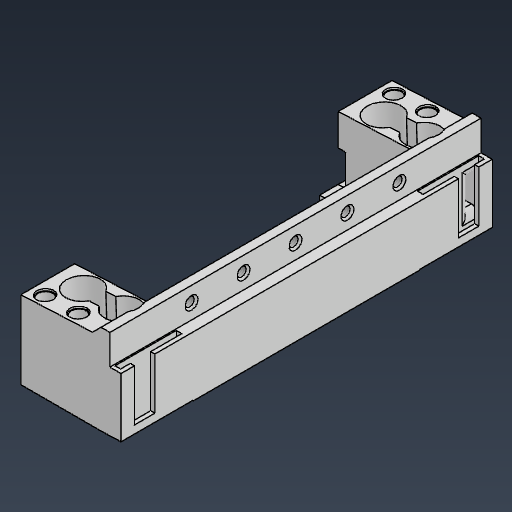
# Autodesk Inventor part: FonrtMount
Saved by Autodesk Inventor 2026.2 (Build 302298010, 298A)
## iProperties
Created: 2026-04-04
Part Number: FonrtMount
Material: Generic
Document SubType Name: Modeling
Designer: szymo
Density: 1 g/cm^3
Appearance: Default
Author: szymo
Autodesk Inventor part; units mm, degrees
(part 1 of 2)
ref_plane "YZ Plane" through (0, 0, 0) normal (1, 0, 0) x (0, 1, 0)
ref_plane "XZ Plane" through (0, 0, 0) normal (0, 1, 0) x (-1, 0, 0)
ref_plane "XY Plane" through (0, 0, 0) normal (0, 0, 1) x (1, 0, 0)
sketch "Sketch1" plane through (0, 0, 0) normal (0, 0, 1) x (1, 0, 0)
  line L0 (-27, 86.2958) -> (-6.5, 86.2958) projected
  line L1 (-6.5, 86.2958) -> (-6.5, 69.7958) projected
  line L2 (-27, 69.7958) -> (-6.5, 69.7958) projected
  line L3 (-27, 86.2958) -> (-27, 69.7958) projected
  line L4 (0, 94.9) -> (0, 81.9) projected
  line L5 (0, 81.9) -> (-3, 81.9) projected
  line L6 (-3, 81.9) -> (-3, 89.9) projected
  line L7 (-3, 89.9) -> (-5, 89.9) projected
  line L8 (-5, 89.9) -> (0, 94.9) projected
  circle A0 centre (-14.5, 55.2958) radius 14.5 projected
  line L9 (-8.2042, 86.6958) -> (-6, 86.6958)
  line L10 (-6, 86.6958) -> (-6, 69.2958)
  line L11 (-6, 69.2958) -> (-10.7251, 69.2958)
  line L12 (-4, 65.2958) -> (0, 65.2958)
  line L13 (0, 65.2958) -> (0, 81.4)
  line L14 (0, 81.4) -> (-3, 81.4)
  line L15 (-3, 81.4) -> (-3, 89.5)
  line L16 (-5.4, 89.5) -> (-8.2042, 86.6958)
  line L17 (-5.4, 89.5) -> (-3, 89.5)
  line L18 (-5.4, 89.5) -> (-5, 89.9) construction
  line L19 (-9.2085, 69.2958) -> (-9.2085, 68.7958)
  line L20 (-7.7042, 87.1958) -> (-7.7042, 86.6958)
  arc A1 (-19.3741, 42.1797) -> (-18.7931, 40.8751) centre (-13.6387, 43.9522) ccw construction
  arc A2 (-18.9897, 42.5035) -> (-19.3741, 42.1797) centre (-13, 35.0012) ccw construction
  arc A3 (-17.8029, 41.709) -> (-18.9897, 42.5035) centre (-21.712, 37.1532) ccw construction
  arc A4 (-17.4452, 41.9512) -> (-17.8029, 41.709) centre (-13, 35.0012) ccw construction
  arc A5 (-17.7423, 43.3481) -> (-17.4452, 41.9512) centre (-11.7637, 43.8894) ccw construction
  arc A6 (-17.299, 43.5848) -> (-17.7423, 43.3481) centre (-13, 35.0012) ccw construction
  arc A7 (-16.3033, 42.561) -> (-17.299, 43.5848) centre (-21.0742, 38.9175) ccw construction
  arc A8 (-15.9031, 42.7235) -> (-16.3033, 42.561) centre (-13, 35.0012) ccw construction
  arc A9 (-15.9033, 44.1517) -> (-15.9031, 42.7235) centre (-9.9428, 43.4382) ccw construction
  arc A10 (-15.4204, 44.2911) -> (-15.9033, 44.1517) centre (-13, 35.0012) ccw construction
  arc A11 (-14.6593, 43.0826) -> (-15.4204, 44.2911) centre (-20.0835, 40.5106) ccw construction
  arc A12 (-14.2341, 43.1584) -> (-14.6593, 43.0826) centre (-13, 35.0012) ccw construction
  arc A13 (-13.9373, 44.5553) -> (-14.2341, 43.1584) centre (-8.2554, 42.6182) ccw construction
  arc A14 (-13.436, 44.5913) -> (-13.9373, 44.5553) centre (-13, 35.0012) ccw construction
  arc A15 (-12.9429, 43.251) -> (-13.436, 44.5913) centre (-18.7832, 41.8629) ccw construction
  arc A16 (-12.5112, 43.2367) -> (-12.9429, 43.251) centre (-13, 35.0012) ccw construction
  arc A17 (-11.9304, 44.5414) -> (-12.5112, 43.2367) centre (-6.7755, 41.4653) ccw construction
  arc A18 (-11.4326, 44.4724) -> (-11.9304, 44.5414) centre (-13, 35.0012) ccw construction
  arc A19 (-11.2289, 43.0588) -> (-11.4326, 44.4724) centre (-17.2302, 42.9154) ccw construction
  arc A20 (-10.8096, 42.9551) -> (-11.2289, 43.0588) centre (-13, 35.0012) ccw construction
  arc A21 (-9.9703, 44.1106) -> (-10.8096, 42.9551) centre (-5.5675, 40.0299) ccw construction
  arc A22 (-9.4977, 43.9395) -> (-9.9703, 44.1106) centre (-13, 35.0012) ccw construction
  arc A23 (-9.5923, 42.5145) -> (-9.4977, 43.9395) centre (-15.4923, 43.622) ccw construction
  arc A24 (-9.2038, 42.3259) -> (-9.5923, 42.5145) centre (-13, 35.0012) ccw construction
  arc A25 (-8.1425, 43.2816) -> (-9.2038, 42.3259) centre (-4.6844, 38.3747) ccw construction
  arc A26 (-7.7158, 43.016) -> (-8.1425, 43.2816) centre (-13, 35.0012) ccw construction
  arc A27 (-8.1047, 41.6418) -> (-7.7158, 43.016) centre (-13.6455, 43.9518) ccw construction
  arc A28 (-7.7638, 41.3765) -> (-8.1047, 41.6418) centre (-13, 35.0012) ccw construction
  arc A29 (-6.5271, 42.0907) -> (-7.7638, 41.3765) centre (-4.1648, 36.572) ccw construction
  arc A30 (-6.1649, 41.7423) -> (-6.5271, 42.0907) centre (-13, 35.0012) ccw construction
  arc A31 (-6.831, 40.4789) -> (-6.1649, 41.7423) centre (-11.7705, 43.8904) ccw construction
  arc A32 (-6.5527, 40.1486) -> (-6.831, 40.4789) centre (-13, 35.0012) ccw construction
  arc A33 (-5.1945, 40.59) -> (-6.5527, 40.1486) centre (-4.0312, 34.7008) ccw construction
  arc A34 (-4.9127, 40.1739) -> (-5.1945, 40.59) centre (-13, 35.0012) ccw construction
  arc A35 (-5.8269, 39.0766) -> (-4.9127, 40.1739) centre (-9.9492, 43.4405) ccw construction
  arc A36 (-5.6234, 38.6956) -> (-5.8269, 39.0766) centre (-13, 35.0012) ccw construction
  arc A37 (-4.2031, 38.845) -> (-5.6234, 38.6956) centre (-4.2897, 32.8426) ccw construction
  arc A38 (-4.014, 38.3794) -> (-4.2031, 38.845) centre (-13, 35.0012) ccw construction
  arc A39 (-5.1363, 37.4962) -> (-4.014, 38.3794) centre (-8.2612, 42.6218) ccw construction
  arc A40 (-5.0165, 37.0812) -> (-5.1363, 37.4962) centre (-13, 35.0012) ccw construction
  arc A41 (-3.5962, 36.9321) -> (-5.0165, 37.0812) centre (-4.9288, 31.0788) ccw construction
  arc A42 (-3.508, 36.4373) -> (-3.5962, 36.9321) centre (-13, 35.0012) ccw construction
  arc A43 (-4.7894, 35.8067) -> (-3.508, 36.4373) centre (-6.7804, 41.47) ccw construction
  arc A44 (-4.7585, 35.3759) -> (-4.7894, 35.8067) centre (-13, 35.0012) ccw construction
  arc A45 (-3.4002, 34.9347) -> (-4.7585, 35.3759) centre (-5.9207, 29.4864) ccw construction
  arc A46 (-3.4169, 34.4324) -> (-3.4002, 34.9347) centre (-13, 35.0012) ccw construction
  arc A47 (-4.8014, 34.082) -> (-3.4169, 34.4324) centre (-5.5713, 40.0355) ccw construction
  arc A48 (-4.8607, 33.6542) -> (-4.8014, 34.082) centre (-13, 35.0012) ccw construction
  arc A49 (-3.6238, 32.9403) -> (-4.8607, 33.6542) centre (-7.222, 28.1351) ccw construction
  arc A50 (-3.7445, 32.4524) -> (-3.6238, 32.9403) centre (-13, 35.0012) ccw construction
  arc A51 (-5.1716, 32.3975) -> (-3.7445, 32.4524) centre (-4.687, 38.381) ccw construction
  arc A52 (-5.3186, 31.9914) -> (-5.1716, 32.3975) centre (-13, 35.0012) ccw construction
  arc A53 (-4.2572, 31.0359) -> (-5.3186, 31.9914) centre (-8.7758, 27.0838) ccw construction
  arc A54 (-4.4767, 30.5838) -> (-4.2572, 31.0359) centre (-13, 35.0012) ccw construction
  arc A55 (-5.884, 30.8268) -> (-4.4767, 30.5838) centre (-4.1659, 36.5788) ccw construction
  arc A56 (-6.1122, 30.4601) -> (-5.884, 30.8268) centre (-13, 35.0012) ccw construction
  arc A57 (-5.2727, 29.3048) -> (-6.1122, 30.4601) centre (-10.5142, 26.3786) ccw construction
  arc A58 (-5.5814, 28.9082) -> (-5.2727, 29.3048) centre (-13, 35.0012) ccw construction
  arc A59 (-6.9074, 29.4385) -> (-5.5814, 28.9082) centre (-4.031, 34.7076) ccw construction
  arc A60 (-7.2069, 29.1273) -> (-6.9074, 29.4385) centre (-13, 35.0012) ccw construction
  arc A61 (-6.6259, 27.8227) -> (-7.2069, 29.1273) centre (-12.3613, 26.0502) ccw construction
  arc A62 (-7.0103, 27.4989) -> (-6.6259, 27.8227) centre (-13, 35.0012) ccw construction
  arc A63 (-8.1971, 28.2934) -> (-7.0103, 27.4989) centre (-4.288, 32.8492) ccw construction
  arc A64 (-8.5548, 28.0512) -> (-8.1971, 28.2934) centre (-13, 35.0012) ccw construction
  arc A65 (-8.2577, 26.6543) -> (-8.5548, 28.0512) centre (-14.2363, 26.113) ccw construction
  arc A66 (-8.701, 26.4176) -> (-8.2577, 26.6543) centre (-13, 35.0012) ccw construction
  arc A67 (-9.6967, 27.4414) -> (-8.701, 26.4176) centre (-4.9258, 31.0849) ccw construction
  arc A68 (-10.0969, 27.2789) -> (-9.6967, 27.4414) centre (-13, 35.0012) ccw construction
  arc A69 (-10.0967, 25.8507) -> (-10.0969, 27.2789) centre (-16.0572, 26.5642) ccw construction
  arc A70 (-10.5796, 25.7113) -> (-10.0967, 25.8507) centre (-13, 35.0012) ccw construction
  arc A71 (-11.3407, 26.9198) -> (-10.5796, 25.7113) centre (-5.9165, 29.4918) ccw construction
  arc A72 (-11.7659, 26.844) -> (-11.3407, 26.9198) centre (-13, 35.0012) ccw construction
  arc A73 (-12.0627, 25.4471) -> (-11.7659, 26.844) centre (-17.7446, 27.3842) ccw construction
  arc A74 (-12.564, 25.4111) -> (-12.0627, 25.4471) centre (-13, 35.0012) ccw construction
  arc A75 (-13.0571, 26.7514) -> (-12.564, 25.4111) centre (-7.2168, 28.1395) ccw construction
  arc A76 (-13.4888, 26.7657) -> (-13.0571, 26.7514) centre (-13, 35.0012) ccw construction
  arc A77 (-14.0696, 25.461) -> (-13.4888, 26.7657) centre (-19.2245, 28.5371) ccw construction
  arc A78 (-14.5674, 25.53) -> (-14.0696, 25.461) centre (-13, 35.0012) ccw construction
  arc A79 (-14.7711, 26.9436) -> (-14.5674, 25.53) centre (-8.7698, 27.087) ccw construction
  arc A80 (-15.1904, 27.0473) -> (-14.7711, 26.9436) centre (-13, 35.0012) ccw construction
  arc A81 (-16.0297, 25.8918) -> (-15.1904, 27.0473) centre (-20.4325, 29.9725) ccw construction
  arc A82 (-16.5023, 26.0629) -> (-16.0297, 25.8918) centre (-13, 35.0012) ccw construction
  arc A83 (-16.4077, 27.4879) -> (-16.5023, 26.0629) centre (-10.5077, 26.3804) ccw construction
  arc A84 (-16.7962, 27.6765) -> (-16.4077, 27.4879) centre (-13, 35.0012) ccw construction
  arc A85 (-17.8575, 26.7208) -> (-16.7962, 27.6765) centre (-21.3156, 31.6277) ccw construction
  arc A86 (-18.2842, 26.9864) -> (-17.8575, 26.7208) centre (-13, 35.0012) ccw construction
  arc A87 (-17.8953, 28.3605) -> (-18.2842, 26.9864) centre (-12.3545, 26.0506) ccw construction
  arc A88 (-18.2362, 28.6259) -> (-17.8953, 28.3605) centre (-13, 35.0012) ccw construction
  arc A89 (-19.4729, 27.9117) -> (-18.2362, 28.6259) centre (-21.8352, 33.4304) ccw construction
  arc A90 (-19.8351, 28.2601) -> (-19.4729, 27.9117) centre (-13, 35.0012) ccw construction
  arc A91 (-19.169, 29.5235) -> (-19.8351, 28.2601) centre (-14.2295, 26.112) ccw construction
  arc A92 (-19.4473, 29.8538) -> (-19.169, 29.5235) centre (-13, 35.0012) ccw construction
  arc A93 (-20.8055, 29.4124) -> (-19.4473, 29.8538) centre (-21.9688, 35.3016) ccw construction
  arc A94 (-21.0873, 29.8285) -> (-20.8055, 29.4124) centre (-13, 35.0012) ccw construction
  arc A95 (-20.1731, 30.9258) -> (-21.0873, 29.8285) centre (-16.0508, 26.5619) ccw construction
  arc A96 (-20.3766, 31.3068) -> (-20.1731, 30.9258) centre (-13, 35.0012) ccw construction
  arc A97 (-21.7969, 31.1574) -> (-20.3766, 31.3068) centre (-21.7103, 37.1598) ccw construction
  arc A98 (-21.986, 31.623) -> (-21.7969, 31.1574) centre (-13, 35.0012) ccw construction
  arc A99 (-20.8637, 32.5062) -> (-21.986, 31.623) centre (-17.7388, 27.3806) ccw construction
  arc A100 (-20.9835, 32.9212) -> (-20.8637, 32.5062) centre (-13, 35.0012) ccw construction
  arc A101 (-22.4038, 33.0703) -> (-20.9835, 32.9212) centre (-21.0712, 38.9236) ccw construction
  arc A102 (-22.492, 33.5651) -> (-22.4038, 33.0703) centre (-13, 35.0012) ccw construction
  arc A103 (-21.2106, 34.1957) -> (-22.492, 33.5651) centre (-19.2196, 28.5324) ccw construction
  arc A104 (-21.2415, 34.6265) -> (-21.2106, 34.1957) centre (-13, 35.0012) ccw construction
  arc A105 (-22.5998, 35.0677) -> (-21.2415, 34.6265) centre (-20.0793, 40.516) ccw construction
  arc A106 (-22.5831, 35.57) -> (-22.5998, 35.0677) centre (-13, 35.0012) ccw construction
  arc A107 (-21.1986, 35.9204) -> (-22.5831, 35.57) centre (-20.4287, 29.9669) ccw construction
  arc A108 (-21.1393, 36.3482) -> (-21.1986, 35.9204) centre (-13, 35.0012) ccw construction
  arc A109 (-22.3762, 37.0621) -> (-21.1393, 36.3482) centre (-18.778, 41.8673) ccw construction
  arc A110 (-22.2555, 37.55) -> (-22.3762, 37.0621) centre (-13, 35.0012) ccw construction
  arc A111 (-20.8284, 37.6049) -> (-22.2555, 37.55) centre (-21.313, 31.6214) ccw construction
  arc A112 (-20.6814, 38.011) -> (-20.8284, 37.6049) centre (-13, 35.0012) ccw construction
  arc A113 (-21.7428, 38.9665) -> (-20.6814, 38.011) centre (-17.2242, 42.9186) ccw construction
  arc A114 (-21.5233, 39.4186) -> (-21.7428, 38.9665) centre (-13, 35.0012) ccw construction
  arc A115 (-20.116, 39.1756) -> (-21.5233, 39.4186) centre (-21.8341, 33.4236) ccw construction
  arc A116 (-19.8878, 39.5423) -> (-20.116, 39.1756) centre (-13, 35.0012) ccw construction
  arc A117 (-20.7273, 40.6976) -> (-19.8878, 39.5423) centre (-15.4858, 43.6238) ccw construction
  arc A118 (-20.4186, 41.0942) -> (-20.7273, 40.6976) centre (-13, 35.0012) ccw construction
  arc A119 (-19.0926, 40.5639) -> (-20.4186, 41.0942) centre (-21.969, 35.2948) ccw construction
  arc A120 (-18.7931, 40.8751) -> (-19.0926, 40.5639) centre (-13, 35.0012) ccw construction
  circle A121 centre (-13, 35.0012) radius 9.6 construction
  line L21 (-4, 65.2958) -> (-27, 65.2958)
  line L22 (-27, 65.2958) -> (-27, 24.2538) construction
  line L23 (-27, 65.2958) -> (-27, 69.2958)
  line L24 (-27, 69.2958) -> (-9.2085, 69.2958)
  point P0 (0, 0)
  dimension "d0" = 4.5
  dimension "d1" = 0.5
  dimension "d2" = 0.5
  dimension "d3" = 0.4
  dimension "d4" = 45
  dimension "d5" = 0.4
  dimension "d6" = 0.5
  dimension "d11" = 0.5
  dimension "d12" = 0.5
  dimension "d32" = 2
  constraints: 32 end point, 7 perpendicular, 4 point on line, 3 horizontal, 3 point on circle, 3 vertical, 2 collinear, 1 coincident, 1 tangent, 3 other
  measures "d0" distance between parallel lines of L12 L2
  measures "d1" distance between parallel lines of L2 L11
  measures "d2" distance between parallel lines of L1 L10
  measures "d3" distance between parallel lines of L9 L0
  measures "d4" angle of L9 L16
  measures "d5" distance between parallel lines of L7 L17
  measures "d6" distance between parallel lines of L5 L14
  measures "d11" distance of L19.start L19.end
  measures "d12" distance of L20.start L20.end
  measures "d32" distance edge to line of A0 L22
extrude "Extrusion2" add sketch "Sketch1" along normal blind 19 and the other way blind 18.4 contours L19 L11 L10 L9 L20 L16 L17 L6 L15 L14 L13 L12 A0
sketch "Sketch2" plane through (0, 0, -18.4) normal (0, 0, -1) x (-1, 0, 0)
  arc A0 (18.7931, 40.8751) -> (19.3741, 42.1797) centre (13.6387, 43.9522) ccw construction
  arc A1 (19.3741, 42.1797) -> (18.9897, 42.5035) centre (13, 35.0012) ccw construction
  arc A2 (18.9897, 42.5035) -> (17.8029, 41.709) centre (21.712, 37.1532) ccw construction
  arc A3 (17.8029, 41.709) -> (17.4452, 41.9512) centre (13, 35.0012) ccw construction
  arc A4 (17.4452, 41.9512) -> (17.7423, 43.3481) centre (11.7637, 43.8894) ccw construction
  arc A5 (17.7423, 43.3481) -> (17.299, 43.5848) centre (13, 35.0012) ccw construction
  arc A6 (17.299, 43.5848) -> (16.3033, 42.561) centre (21.0742, 38.9175) ccw construction
  arc A7 (16.3033, 42.561) -> (15.9031, 42.7235) centre (13, 35.0012) ccw construction
  arc A8 (15.9031, 42.7235) -> (15.9033, 44.1517) centre (9.9428, 43.4382) ccw construction
  arc A9 (15.9033, 44.1517) -> (15.4204, 44.2911) centre (13, 35.0012) ccw construction
  arc A10 (15.4204, 44.2911) -> (14.6593, 43.0826) centre (20.0835, 40.5106) ccw construction
  arc A11 (14.6593, 43.0826) -> (14.2341, 43.1584) centre (13, 35.0012) ccw construction
  arc A12 (14.2341, 43.1584) -> (13.9373, 44.5553) centre (8.2554, 42.6182) ccw construction
  arc A13 (13.9373, 44.5553) -> (13.436, 44.5913) centre (13, 35.0012) ccw construction
  arc A14 (13.436, 44.5913) -> (12.9429, 43.251) centre (18.7832, 41.8629) ccw construction
  arc A15 (12.9429, 43.251) -> (12.5112, 43.2367) centre (13, 35.0012) ccw construction
  arc A16 (12.5112, 43.2367) -> (11.9304, 44.5414) centre (6.7755, 41.4653) ccw construction
  arc A17 (11.9304, 44.5414) -> (11.4326, 44.4724) centre (13, 35.0012) ccw construction
  arc A18 (11.4326, 44.4724) -> (11.2289, 43.0588) centre (17.2302, 42.9154) ccw construction
  arc A19 (11.2289, 43.0588) -> (10.8096, 42.9551) centre (13, 35.0012) ccw construction
  arc A20 (10.8096, 42.9551) -> (9.9703, 44.1106) centre (5.5675, 40.0299) ccw construction
  arc A21 (9.9703, 44.1106) -> (9.4977, 43.9395) centre (13, 35.0012) ccw construction
  arc A22 (9.4977, 43.9395) -> (9.5923, 42.5145) centre (15.4923, 43.622) ccw construction
  arc A23 (9.5923, 42.5145) -> (9.2038, 42.3259) centre (13, 35.0012) ccw construction
  arc A24 (9.2038, 42.3259) -> (8.1425, 43.2816) centre (4.6844, 38.3747) ccw construction
  arc A25 (8.1425, 43.2816) -> (7.7158, 43.016) centre (13, 35.0012) ccw construction
  arc A26 (7.7158, 43.016) -> (8.1047, 41.6418) centre (13.6455, 43.9518) ccw construction
  arc A27 (8.1047, 41.6418) -> (7.7638, 41.3765) centre (13, 35.0012) ccw construction
  arc A28 (7.7638, 41.3765) -> (6.5271, 42.0907) centre (4.1648, 36.572) ccw construction
  arc A29 (6.5271, 42.0907) -> (6.1649, 41.7423) centre (13, 35.0012) ccw construction
  arc A30 (6.1649, 41.7423) -> (6.831, 40.4789) centre (11.7705, 43.8904) ccw construction
  arc A31 (6.831, 40.4789) -> (6.5527, 40.1486) centre (13, 35.0012) ccw construction
  arc A32 (6.5527, 40.1486) -> (5.1945, 40.59) centre (4.0312, 34.7008) ccw construction
  arc A33 (5.1945, 40.59) -> (4.9127, 40.1739) centre (13, 35.0012) ccw construction
  arc A34 (4.9127, 40.1739) -> (5.8269, 39.0766) centre (9.9492, 43.4405) ccw construction
  arc A35 (5.8269, 39.0766) -> (5.6234, 38.6956) centre (13, 35.0012) ccw construction
  arc A36 (5.6234, 38.6956) -> (4.2031, 38.845) centre (4.2897, 32.8426) ccw construction
  arc A37 (4.2031, 38.845) -> (4.014, 38.3794) centre (13, 35.0012) ccw construction
  arc A38 (4.014, 38.3794) -> (5.1363, 37.4962) centre (8.2612, 42.6218) ccw construction
  arc A39 (5.1363, 37.4962) -> (5.0165, 37.0812) centre (13, 35.0012) ccw construction
  arc A40 (5.0165, 37.0812) -> (3.5962, 36.9321) centre (4.9288, 31.0788) ccw construction
  arc A41 (3.5962, 36.9321) -> (3.508, 36.4373) centre (13, 35.0012) ccw construction
  arc A42 (3.508, 36.4373) -> (4.7894, 35.8067) centre (6.7804, 41.47) ccw construction
  arc A43 (4.7894, 35.8067) -> (4.7585, 35.3759) centre (13, 35.0012) ccw construction
  arc A44 (4.7585, 35.3759) -> (3.4002, 34.9347) centre (5.9207, 29.4864) ccw construction
  arc A45 (3.4002, 34.9347) -> (3.4169, 34.4324) centre (13, 35.0012) ccw construction
  arc A46 (3.4169, 34.4324) -> (4.8014, 34.082) centre (5.5713, 40.0355) ccw construction
  arc A47 (4.8014, 34.082) -> (4.8607, 33.6542) centre (13, 35.0012) ccw construction
  arc A48 (4.8607, 33.6542) -> (3.6238, 32.9403) centre (7.222, 28.1351) ccw construction
  arc A49 (3.6238, 32.9403) -> (3.7445, 32.4524) centre (13, 35.0012) ccw construction
  arc A50 (3.7445, 32.4524) -> (5.1716, 32.3975) centre (4.687, 38.381) ccw construction
  arc A51 (5.1716, 32.3975) -> (5.3186, 31.9914) centre (13, 35.0012) ccw construction
  arc A52 (5.3186, 31.9914) -> (4.2572, 31.0359) centre (8.7758, 27.0838) ccw construction
  arc A53 (4.2572, 31.0359) -> (4.4767, 30.5838) centre (13, 35.0012) ccw construction
  arc A54 (4.4767, 30.5838) -> (5.884, 30.8268) centre (4.1659, 36.5788) ccw construction
  arc A55 (5.884, 30.8268) -> (6.1122, 30.4601) centre (13, 35.0012) ccw construction
  arc A56 (6.1122, 30.4601) -> (5.2727, 29.3048) centre (10.5142, 26.3786) ccw construction
  arc A57 (5.2727, 29.3048) -> (5.5814, 28.9082) centre (13, 35.0012) ccw construction
  arc A58 (5.5814, 28.9082) -> (6.9074, 29.4385) centre (4.031, 34.7076) ccw construction
  arc A59 (6.9074, 29.4385) -> (7.2069, 29.1273) centre (13, 35.0012) ccw construction
  arc A60 (7.2069, 29.1273) -> (6.6259, 27.8227) centre (12.3613, 26.0502) ccw construction
  arc A61 (6.6259, 27.8227) -> (7.0103, 27.4989) centre (13, 35.0012) ccw construction
  arc A62 (7.0103, 27.4989) -> (8.1971, 28.2934) centre (4.288, 32.8492) ccw construction
  arc A63 (8.1971, 28.2934) -> (8.5548, 28.0512) centre (13, 35.0012) ccw construction
  arc A64 (8.5548, 28.0512) -> (8.2577, 26.6543) centre (14.2363, 26.113) ccw construction
  arc A65 (8.2577, 26.6543) -> (8.701, 26.4176) centre (13, 35.0012) ccw construction
  arc A66 (8.701, 26.4176) -> (9.6967, 27.4414) centre (4.9258, 31.0849) ccw construction
  arc A67 (9.6967, 27.4414) -> (10.0969, 27.2789) centre (13, 35.0012) ccw construction
  arc A68 (10.0969, 27.2789) -> (10.0967, 25.8507) centre (16.0572, 26.5642) ccw construction
  arc A69 (10.0967, 25.8507) -> (10.5796, 25.7113) centre (13, 35.0012) ccw construction
  arc A70 (10.5796, 25.7113) -> (11.3407, 26.9198) centre (5.9165, 29.4918) ccw construction
  arc A71 (11.3407, 26.9198) -> (11.7659, 26.844) centre (13, 35.0012) ccw construction
  arc A72 (11.7659, 26.844) -> (12.0627, 25.4471) centre (17.7446, 27.3842) ccw construction
  arc A73 (12.0627, 25.4471) -> (12.564, 25.4111) centre (13, 35.0012) ccw construction
  arc A74 (12.564, 25.4111) -> (13.0571, 26.7514) centre (7.2168, 28.1395) ccw construction
  arc A75 (13.0571, 26.7514) -> (13.4888, 26.7657) centre (13, 35.0012) ccw construction
  arc A76 (13.4888, 26.7657) -> (14.0696, 25.461) centre (19.2245, 28.5371) ccw construction
  arc A77 (14.0696, 25.461) -> (14.5674, 25.53) centre (13, 35.0012) ccw construction
  arc A78 (14.5674, 25.53) -> (14.7711, 26.9436) centre (8.7698, 27.087) ccw construction
  arc A79 (14.7711, 26.9436) -> (15.1904, 27.0473) centre (13, 35.0012) ccw construction
  arc A80 (15.1904, 27.0473) -> (16.0297, 25.8918) centre (20.4325, 29.9725) ccw construction
  arc A81 (16.0297, 25.8918) -> (16.5023, 26.0629) centre (13, 35.0012) ccw construction
  arc A82 (16.5023, 26.0629) -> (16.4077, 27.4879) centre (10.5077, 26.3804) ccw construction
  arc A83 (16.4077, 27.4879) -> (16.7962, 27.6765) centre (13, 35.0012) ccw construction
  arc A84 (16.7962, 27.6765) -> (17.8575, 26.7208) centre (21.3156, 31.6277) ccw construction
  arc A85 (17.8575, 26.7208) -> (18.2842, 26.9864) centre (13, 35.0012) ccw construction
  arc A86 (18.2842, 26.9864) -> (17.8953, 28.3605) centre (12.3545, 26.0506) ccw construction
  arc A87 (17.8953, 28.3605) -> (18.2362, 28.6259) centre (13, 35.0012) ccw construction
  arc A88 (18.2362, 28.6259) -> (19.4729, 27.9117) centre (21.8352, 33.4304) ccw construction
  arc A89 (19.4729, 27.9117) -> (19.8351, 28.2601) centre (13, 35.0012) ccw construction
  arc A90 (19.8351, 28.2601) -> (19.169, 29.5235) centre (14.2295, 26.112) ccw construction
  arc A91 (19.169, 29.5235) -> (19.4473, 29.8538) centre (13, 35.0012) ccw construction
  arc A92 (19.4473, 29.8538) -> (20.8055, 29.4124) centre (21.9688, 35.3016) ccw construction
  arc A93 (20.8055, 29.4124) -> (21.0873, 29.8285) centre (13, 35.0012) ccw construction
  arc A94 (21.0873, 29.8285) -> (20.1731, 30.9258) centre (16.0508, 26.5619) ccw construction
  arc A95 (20.1731, 30.9258) -> (20.3766, 31.3068) centre (13, 35.0012) ccw construction
  arc A96 (20.3766, 31.3068) -> (21.7969, 31.1574) centre (21.7103, 37.1598) ccw construction
  arc A97 (21.7969, 31.1574) -> (21.986, 31.623) centre (13, 35.0012) ccw construction
  arc A98 (21.986, 31.623) -> (20.8637, 32.5062) centre (17.7388, 27.3806) ccw construction
  arc A99 (20.8637, 32.5062) -> (20.9835, 32.9212) centre (13, 35.0012) ccw construction
  arc A100 (20.9835, 32.9212) -> (22.4038, 33.0703) centre (21.0712, 38.9236) ccw construction
  arc A101 (22.4038, 33.0703) -> (22.492, 33.5651) centre (13, 35.0012) ccw construction
  arc A102 (22.492, 33.5651) -> (21.2106, 34.1957) centre (19.2196, 28.5324) ccw construction
  arc A103 (21.2106, 34.1957) -> (21.2415, 34.6265) centre (13, 35.0012) ccw construction
  arc A104 (21.2415, 34.6265) -> (22.5998, 35.0677) centre (20.0793, 40.516) ccw construction
  arc A105 (22.5998, 35.0677) -> (22.5831, 35.57) centre (13, 35.0012) ccw construction
  arc A106 (22.5831, 35.57) -> (21.1986, 35.9204) centre (20.4287, 29.9669) ccw construction
  arc A107 (21.1986, 35.9204) -> (21.1393, 36.3482) centre (13, 35.0012) ccw construction
  arc A108 (21.1393, 36.3482) -> (22.3762, 37.0621) centre (18.778, 41.8673) ccw construction
  arc A109 (22.3762, 37.0621) -> (22.2555, 37.55) centre (13, 35.0012) ccw construction
  arc A110 (22.2555, 37.55) -> (20.8284, 37.6049) centre (21.313, 31.6214) ccw construction
  arc A111 (20.8284, 37.6049) -> (20.6814, 38.011) centre (13, 35.0012) ccw construction
  arc A112 (20.6814, 38.011) -> (21.7428, 38.9665) centre (17.2242, 42.9186) ccw construction
  arc A113 (21.7428, 38.9665) -> (21.5233, 39.4186) centre (13, 35.0012) ccw construction
  arc A114 (21.5233, 39.4186) -> (20.116, 39.1756) centre (21.8341, 33.4236) ccw construction
  arc A115 (20.116, 39.1756) -> (19.8878, 39.5423) centre (13, 35.0012) ccw construction
  arc A116 (19.8878, 39.5423) -> (20.7273, 40.6976) centre (15.4858, 43.6238) ccw construction
  arc A117 (20.7273, 40.6976) -> (20.4186, 41.0942) centre (13, 35.0012) ccw construction
  arc A118 (20.4186, 41.0942) -> (19.0926, 40.5639) centre (21.969, 35.2948) ccw construction
  arc A119 (19.0926, 40.5639) -> (18.7931, 40.8751) centre (13, 35.0012) ccw construction
  circle A120 centre (13, 35.0012) radius 9.6 construction
  line L0 (23.8, 32.6031) -> (23.8, 65.2958) construction
  line L1 (9.2085, 69.2958) -> (6, 69.2958) projected
  line L2 (6, 69.2958) -> (6, 86.6958) projected
  line L3 (6, 86.6958) -> (7.7042, 86.6958) projected
  line L4 (7.7042, 86.6958) -> (7.7042, 87.1958) projected
  line L5 (7.7042, 87.1958) -> (5.4, 89.5) projected
  line L6 (5.4, 89.5) -> (3, 89.5) projected
  line L7 (3, 89.5) -> (3, 81.4) projected
  line L8 (3, 81.4) -> (0, 81.4) projected
  line L9 (0, 81.4) -> (0, 65.2958) projected
  line L10 (0, 65.2958) -> (4, 65.2958) projected
  arc A121 (9.2085, 68.7958) -> (4, 65.2958) centre (14.5, 55.2958) ccw projected
  line L11 (9.2085, 68.7958) -> (9.2085, 69.2958) projected
  line L12 (4, 65.2958) -> (23.8, 65.2958)
  line L13 (23.8, 65.2958) -> (23.8, 69.2958)
  line L14 (23.8, 69.2958) -> (9.2085, 69.2958)
  circle A122 centre (14.5, 55.2958) radius 14.5 projected
  point P0 (0, 0)
  dimension "d33" = 5.2
  dimension "d35" = 1.2
  constraints: 8 end point, 2 vertical, 1 coincident, 1 horizontal, 1 perpendicular, 3 other
  measures "d33" distance edge to line of A122 L0
extrude "Extrusion3" add sketch "Sketch2" along normal blind 17.1 contours L11 A121 L10 L9 L8 L7 L6 L5 L4 L3 L2 L1 | L14 A122 L11 | A122 L14 L13 L12 A121 | L14 L13 A122
sketch "Sketch3" plane through (0, 0, 19) normal (0, 0, 1) x (1, 0, 0)
  arc A0 (-9.6825, 42.5548) -> (-9.605, 43.9808) centre (-15.5954, 43.5915) ccw construction
  arc A1 (-9.605, 43.9808) -> (-10.0796, 44.1462) centre (-13, 35.0012) ccw construction
  arc A2 (-10.0796, 44.1462) -> (-10.905, 42.9808) centre (-5.6283, 40.1185) ccw construction
  arc A3 (-10.905, 42.9808) -> (-11.3255, 43.0795) centre (-13, 35.0012) ccw construction
  arc A4 (-11.3255, 43.0795) -> (-11.5461, 44.4905) centre (-17.3247, 42.8642) ccw construction
  arc A5 (-11.5461, 44.4905) -> (-12.0447, 44.5536) centre (-13, 35.0012) ccw construction
  arc A6 (-12.0447, 44.5536) -> (-12.6098, 43.242) centre (-6.8533, 41.5393) ccw construction
  arc A7 (-12.6098, 43.242) -> (-13.0416, 43.2511) centre (-13, 35.0012) ccw construction
  arc A8 (-13.0416, 43.2511) -> (-13.5508, 44.5854) centre (-18.865, 41.7932) ccw construction
  arc A9 (-13.5508, 44.5854) -> (-14.0517, 44.5434) centre (-13, 35.0012) ccw construction
  arc A10 (-14.0517, 44.5434) -> (-14.3317, 43.143) centre (-8.347, 42.6744) ccw construction
  arc A11 (-14.3317, 43.143) -> (-14.756, 43.0622) centre (-13, 35.0012) ccw construction
  arc A12 (-14.756, 43.0622) -> (-15.5314, 44.2614) centre (-20.1489, 40.4254) ccw construction
  arc A13 (-15.5314, 44.2614) -> (-16.0126, 44.1162) centre (-13, 35.0012) ccw construction
  arc A14 (-16.0126, 44.1162) -> (-15.9954, 42.6882) centre (-10.044, 43.4742) ccw construction
  arc A15 (-15.9954, 42.6882) -> (-16.3936, 42.5209) centre (-13, 35.0012) ccw construction
  arc A16 (-16.3936, 42.5209) -> (-17.4014, 43.5327) centre (-21.1205, 38.8205) ccw construction
  arc A17 (-17.4014, 43.5327) -> (-17.8419, 43.2907) centre (-13, 35.0012) ccw construction
  arc A18 (-17.8419, 43.2907) -> (-17.5281, 41.8975) centre (-11.8702, 43.9036) ccw construction
  arc A19 (-17.5281, 41.8975) -> (-17.8829, 41.651) centre (-13, 35.0012) ccw construction
  arc A20 (-17.8829, 41.651) -> (-19.0791, 42.4312) centre (-21.7371, 37.0487) ccw construction
  arc A21 (-19.0791, 42.4312) -> (-19.4596, 42.1029) centre (-13, 35.0012) ccw construction
  arc A22 (-19.4596, 42.1029) -> (-18.863, 40.8053) centre (-13.7458, 43.944) ccw construction
  arc A23 (-18.863, 40.8053) -> (-19.1587, 40.4905) centre (-13, 35.0012) ccw construction
  arc A24 (-19.1587, 40.4905) -> (-20.491, 41.0049) centre (-21.9719, 35.1874) ccw construction
  arc A25 (-20.491, 41.0049) -> (-20.795, 40.6047) centre (-13, 35.0012) ccw construction
  arc A26 (-20.795, 40.6047) -> (-19.9416, 39.4595) centre (-15.5888, 43.5935) ccw construction
  arc A27 (-19.9416, 39.4595) -> (-20.1654, 39.0901) centre (-13, 35.0012) ccw construction
  arc A28 (-20.1654, 39.0901) -> (-21.5756, 39.3163) centre (-21.8145, 33.318) ccw construction
  arc A29 (-21.5756, 39.3163) -> (-21.7896, 38.8615) centre (-13, 35.0012) ccw construction
  arc A30 (-21.7896, 38.8615) -> (-20.7169, 37.9188) centre (-17.3187, 42.8675) ccw construction
  arc A31 (-20.7169, 37.9188) -> (-20.859, 37.5109) centre (-13, 35.0012) ccw construction
  arc A32 (-20.859, 37.5109) -> (-22.2853, 37.439) centre (-21.272, 31.5221) ccw construction
  arc A33 (-22.2853, 37.439) -> (-22.4002, 36.9497) centre (-13, 35.0012) ccw construction
  arc A34 (-22.4002, 36.9497) -> (-21.1548, 36.2506) centre (-18.8598, 41.7976) ccw construction
  arc A35 (-21.1548, 36.2506) -> (-21.2091, 35.8221) centre (-13, 35.0012) ccw construction
  arc A36 (-21.2091, 35.8221) -> (-22.5893, 35.4552) centre (-20.3678, 29.8783) ccw construction
  arc A37 (-22.5893, 35.4552) -> (-22.5999, 34.9527) centre (-13, 35.0012) ccw construction
  arc A38 (-22.5999, 34.9527) -> (-21.2364, 34.5278) centre (-20.1448, 40.4308) ccw construction
  arc A39 (-21.2364, 34.5278) -> (-21.2003, 34.0974) centre (-13, 35.0012) ccw construction
  arc A40 (-21.2003, 34.0974) -> (-22.4741, 33.4516) centre (-19.1417, 28.4584) ccw construction
  arc A41 (-22.4741, 33.4516) -> (-22.38, 32.9579) centre (-13, 35.0012) ccw construction
  arc A42 (-22.38, 32.9579) -> (-20.958, 32.8257) centre (-21.1176, 38.8267) ccw construction
  arc A43 (-20.958, 32.8257) -> (-20.8332, 32.4122) centre (-13, 35.0012) ccw construction
  arc A44 (-20.8332, 32.4122) -> (-21.9449, 31.5157) centre (-17.6472, 27.3244) ccw construction
  arc A45 (-21.9449, 31.5157) -> (-21.7502, 31.0523) centre (-13, 35.0012) ccw construction
  arc A46 (-21.7502, 31.0523) -> (-20.3318, 31.2187) centre (-21.7355, 37.0553) ccw construction
  arc A47 (-20.3318, 31.2187) -> (-20.1238, 30.8402) centre (-13, 35.0012) ccw construction
  arc A48 (-20.1238, 30.8402) -> (-21.0247, 29.7321) centre (-15.9496, 26.526) ccw construction
  arc A49 (-21.0247, 29.7321) -> (-20.738, 29.3193) centre (-13, 35.0012) ccw construction
  arc A50 (-20.738, 29.3193) -> (-19.3852, 29.777) centre (-21.9717, 35.1942) ccw construction
  arc A51 (-19.3852, 29.777) -> (-19.103, 29.45) centre (-13, 35.0012) ccw construction
  arc A52 (-19.103, 29.45) -> (-19.7539, 28.1788) centre (-14.123, 26.0979) ccw construction
  arc A53 (-19.7539, 28.1788) -> (-19.3876, 27.8347) centre (-13, 35.0012) ccw construction
  arc A54 (-19.3876, 27.8347) -> (-18.1595, 28.5636) centre (-21.8158, 33.3247) ccw construction
  arc A55 (-18.1595, 28.5636) -> (-17.8155, 28.3024) centre (-13, 35.0012) ccw construction
  arc A56 (-17.8155, 28.3024) -> (-18.1878, 26.9237) centre (-12.2474, 26.059) ccw construction
  arc A57 (-18.1878, 26.9237) -> (-17.758, 26.6632) centre (-13, 35.0012) ccw construction
  arc A58 (-17.758, 26.6632) -> (-16.7083, 27.6316) centre (-21.2746, 31.5284) ccw construction
  arc A59 (-16.7083, 27.6316) -> (-16.3175, 27.4476) centre (-13, 35.0012) ccw construction
  arc A60 (-16.3175, 27.4476) -> (-16.395, 26.0216) centre (-10.4046, 26.4109) ccw construction
  arc A61 (-16.395, 26.0216) -> (-15.9204, 25.8562) centre (-13, 35.0012) ccw construction
  arc A62 (-15.9204, 25.8562) -> (-15.095, 27.0216) centre (-20.3717, 29.8839) ccw construction
  arc A63 (-15.095, 27.0216) -> (-14.6745, 26.9229) centre (-13, 35.0012) ccw construction
  arc A64 (-14.6745, 26.9229) -> (-14.4539, 25.5119) centre (-8.6753, 27.1382) ccw construction
  arc A65 (-14.4539, 25.5119) -> (-13.9553, 25.4488) centre (-13, 35.0012) ccw construction
  arc A66 (-13.9553, 25.4488) -> (-13.3902, 26.7604) centre (-19.1467, 28.4631) ccw construction
  arc A67 (-13.3902, 26.7604) -> (-12.9584, 26.7513) centre (-13, 35.0012) ccw construction
  arc A68 (-12.9584, 26.7513) -> (-12.4492, 25.417) centre (-7.135, 28.2092) ccw construction
  arc A69 (-12.4492, 25.417) -> (-11.9483, 25.459) centre (-13, 35.0012) ccw construction
  arc A70 (-11.9483, 25.459) -> (-11.6683, 26.8594) centre (-17.653, 27.328) ccw construction
  arc A71 (-11.6683, 26.8594) -> (-11.244, 26.9402) centre (-13, 35.0012) ccw construction
  arc A72 (-11.244, 26.9402) -> (-10.4686, 25.741) centre (-5.8511, 29.577) ccw construction
  arc A73 (-10.4686, 25.741) -> (-9.9874, 25.8861) centre (-13, 35.0012) ccw construction
  arc A74 (-9.9874, 25.8861) -> (-10.0046, 27.3142) centre (-15.956, 26.5282) ccw construction
  arc A75 (-10.0046, 27.3142) -> (-9.6064, 27.4815) centre (-13, 35.0012) ccw construction
  arc A76 (-9.6064, 27.4815) -> (-8.5986, 26.4696) centre (-4.8795, 31.1819) ccw construction
  arc A77 (-8.5986, 26.4696) -> (-8.1581, 26.7117) centre (-13, 35.0012) ccw construction
  arc A78 (-8.1581, 26.7117) -> (-8.4719, 28.1049) centre (-14.1298, 26.0988) ccw construction
  arc A79 (-8.4719, 28.1049) -> (-8.1171, 28.3514) centre (-13, 35.0012) ccw construction
  arc A80 (-8.1171, 28.3514) -> (-6.9209, 27.5712) centre (-4.2629, 32.9537) ccw construction
  arc A81 (-6.9209, 27.5712) -> (-6.5404, 27.8995) centre (-13, 35.0012) ccw construction
  arc A82 (-6.5404, 27.8995) -> (-7.137, 29.1971) centre (-12.2542, 26.0584) ccw construction
  arc A83 (-7.137, 29.1971) -> (-6.8413, 29.5119) centre (-13, 35.0012) ccw construction
  arc A84 (-6.8413, 29.5119) -> (-5.509, 28.9975) centre (-4.0281, 34.815) ccw construction
  arc A85 (-5.509, 28.9975) -> (-5.205, 29.3977) centre (-13, 35.0012) ccw construction
  arc A86 (-5.205, 29.3977) -> (-6.0584, 30.5429) centre (-10.4112, 26.4089) ccw construction
  arc A87 (-6.0584, 30.5429) -> (-5.8346, 30.9123) centre (-13, 35.0012) ccw construction
  arc A88 (-5.8346, 30.9123) -> (-4.4244, 30.6861) centre (-4.1855, 36.6844) ccw construction
  arc A89 (-4.4244, 30.6861) -> (-4.2104, 31.1409) centre (-13, 35.0012) ccw construction
  arc A90 (-4.2104, 31.1409) -> (-5.2831, 32.0836) centre (-8.6813, 27.1349) ccw construction
  arc A91 (-5.2831, 32.0836) -> (-5.141, 32.4915) centre (-13, 35.0012) ccw construction
  arc A92 (-5.141, 32.4915) -> (-3.7147, 32.5634) centre (-4.728, 38.4803) ccw construction
  arc A93 (-3.7147, 32.5634) -> (-3.5998, 33.0527) centre (-13, 35.0012) ccw construction
  arc A94 (-3.5998, 33.0527) -> (-4.8452, 33.7518) centre (-7.1402, 28.2047) ccw construction
  arc A95 (-4.8452, 33.7518) -> (-4.7909, 34.1803) centre (-13, 35.0012) ccw construction
  arc A96 (-4.7909, 34.1803) -> (-3.4107, 34.5472) centre (-5.6322, 40.1241) ccw construction
  arc A97 (-3.4107, 34.5472) -> (-3.4001, 35.0497) centre (-13, 35.0012) ccw construction
  arc A98 (-3.4001, 35.0497) -> (-4.7636, 35.4746) centre (-5.8552, 29.5716) ccw construction
  arc A99 (-4.7636, 35.4746) -> (-4.7997, 35.905) centre (-13, 35.0012) ccw construction
  arc A100 (-4.7997, 35.905) -> (-3.5259, 36.5508) centre (-6.8583, 41.544) ccw construction
  arc A101 (-3.5259, 36.5508) -> (-3.62, 37.0445) centre (-13, 35.0012) ccw construction
  arc A102 (-3.62, 37.0445) -> (-5.042, 37.1767) centre (-4.8824, 31.1757) ccw construction
  arc A103 (-5.042, 37.1767) -> (-5.1668, 37.5902) centre (-13, 35.0012) ccw construction
  arc A104 (-5.1668, 37.5902) -> (-4.0551, 38.4867) centre (-8.3528, 42.678) ccw construction
  arc A105 (-4.0551, 38.4867) -> (-4.2498, 38.9501) centre (-13, 35.0012) ccw construction
  arc A106 (-4.2498, 38.9501) -> (-5.6682, 38.7837) centre (-4.2645, 32.9471) ccw construction
  arc A107 (-5.6682, 38.7837) -> (-5.8762, 39.1622) centre (-13, 35.0012) ccw construction
  arc A108 (-5.8762, 39.1622) -> (-4.9753, 40.2703) centre (-10.0504, 43.4764) ccw construction
  arc A109 (-4.9753, 40.2703) -> (-5.262, 40.6831) centre (-13, 35.0012) ccw construction
  arc A110 (-5.262, 40.6831) -> (-6.6148, 40.2254) centre (-4.0283, 34.8082) ccw construction
  arc A111 (-6.6148, 40.2254) -> (-6.897, 40.5524) centre (-13, 35.0012) ccw construction
  arc A112 (-6.897, 40.5524) -> (-6.2461, 41.8236) centre (-11.877, 43.9045) ccw construction
  arc A113 (-6.2461, 41.8236) -> (-6.6124, 42.1677) centre (-13, 35.0012) ccw construction
  arc A114 (-6.6124, 42.1677) -> (-7.8405, 41.4388) centre (-4.1842, 36.6777) ccw construction
  arc A115 (-7.8405, 41.4388) -> (-8.1845, 41.7) centre (-13, 35.0012) ccw construction
  arc A116 (-8.1845, 41.7) -> (-7.8122, 43.0787) centre (-13.7526, 43.9434) ccw construction
  arc A117 (-7.8122, 43.0787) -> (-8.242, 43.3392) centre (-13, 35.0012) ccw construction
  arc A118 (-8.242, 43.3392) -> (-9.2917, 42.3708) centre (-4.7254, 38.474) ccw construction
  arc A119 (-9.2917, 42.3708) -> (-9.6825, 42.5548) centre (-13, 35.0012) ccw construction
  line L0 (-6, 69.2958) -> (-9.2085, 69.2958) projected
  line L1 (-9.2085, 69.2958) -> (-9.2085, 68.7958) projected
  arc A120 (-4, 65.2958) -> (-9.2085, 68.7958) centre (-14.5, 55.2958) ccw projected
  line L2 (-4, 65.2958) -> (0, 65.2958) projected
  line L3 (0, 65.2958) -> (0, 81.4) projected
  line L4 (0, 81.4) -> (-3, 81.4) projected
  line L5 (-3, 81.4) -> (-3, 89.5) projected
  line L6 (-3, 89.5) -> (-5.4, 89.5) projected
  line L7 (-5.4, 89.5) -> (-7.7042, 87.1958) projected
  line L8 (-7.7042, 87.1958) -> (-7.7042, 86.6958) projected
  line L9 (-7.7042, 86.6958) -> (-6, 86.6958) projected
  line L10 (-6, 86.6958) -> (-6, 69.2958) projected
  circle A121 centre (-13, 35.0012) radius 9.6
  line L11 (-23.8, 30.4052) -> (-23.8, 69.2958)
  line L12 (-23.8, 69.2958) -> (-9.2085, 69.2958)
  line L13 (-4, 65.2958) -> (-23.8, 65.2958) projected
  line L14 (-4, 65.2958) -> (-23.8, 65.2958)
  circle A122 centre (-14.5, 55.2958) radius 14.5 projected
  point P0 (0, 0)
  point P1 (-25.5572, 65.2958)
  dimension "d34" = 5.2
  dimension "d36" = 1.2
  constraints: 6 end point, 2 perpendicular, 1 coincident, 1 vertical, 3 other
  measures "d34" distance edge to line of A122 L11
extrude "Extrusion4" add sketch "Sketch3" along normal blind 16.5 contours L10 L9 L8 L7 L6 L5 L4 L3 L2 A120 L1 L0 | L1 A122 L12 | A120 L13 L11 A122 L12 | A122 L11 L12
sketch "Sketch4" plane through (0, 0, -35.5) normal (0, 0, -1) x (-1, 0, 0)
  line L0 (26.0532, 64.5637) -> (22.0556, 64.7033)
  line L1 (5.4157, 65.2843) -> (22.0556, 64.7033)
  line L2 (5.4157, 65.2843) -> (1.4182, 65.4239)
  line L3 (23.8, 65.2958) -> (23.8, 69.2958)
  line L4 (23.8, 69.2958) -> (6, 69.2958)
  line L5 (6, 69.2958) -> (6, 86.6958)
  line L6 (6, 86.6958) -> (7.7042, 86.6958)
  line L7 (7.7042, 86.6958) -> (7.7042, 87.1958)
  line L8 (7.7042, 87.1958) -> (5.4, 89.5)
  line L9 (5.4, 89.5) -> (3, 89.5)
  line L10 (3, 89.5) -> (3, 81.4)
  line L11 (3, 81.4) -> (0, 81.4)
  line L12 (0, 81.4) -> (0, 65.2958)
  line L13 (0, 65.2958) -> (23.8, 65.2958)
  line L14 (1.4182, 65.4239) -> (0, 65.4735)
  line L15 (27, 52.5631) -> (27, 86.2958)
  line L16 (27, 86.2958) -> (7.7042, 87.1958)
  line L17 (27, 86.2958) -> (6.5, 86.2958)
  line L18 (26.0532, 64.5637) -> (27, 64.5306)
  line L19 (23.8, 65.2958) -> (23.8, 69.2958)
  arc A0 (18.7931, 40.8751) -> (19.3741, 42.1797) centre (13.6387, 43.9522) ccw
  arc A1 (19.3741, 42.1797) -> (18.9897, 42.5035) centre (13, 35.0012) ccw
  arc A2 (18.9897, 42.5035) -> (17.8029, 41.709) centre (21.712, 37.1532) ccw
  arc A3 (17.8029, 41.709) -> (17.4452, 41.9512) centre (13, 35.0012) ccw
  arc A4 (17.4452, 41.9512) -> (17.7423, 43.3481) centre (11.7637, 43.8894) ccw
  arc A5 (17.7423, 43.3481) -> (17.299, 43.5848) centre (13, 35.0012) ccw
  arc A6 (17.299, 43.5848) -> (16.3033, 42.561) centre (21.0742, 38.9175) ccw
  arc A7 (16.3033, 42.561) -> (15.9031, 42.7235) centre (13, 35.0012) ccw
  arc A8 (15.9031, 42.7235) -> (15.9033, 44.1517) centre (9.9428, 43.4382) ccw
  arc A9 (15.9033, 44.1517) -> (15.4204, 44.2911) centre (13, 35.0012) ccw
  arc A10 (15.4204, 44.2911) -> (14.6593, 43.0826) centre (20.0835, 40.5106) ccw
  arc A11 (14.6593, 43.0826) -> (14.2341, 43.1584) centre (13, 35.0012) ccw
  arc A12 (14.2341, 43.1584) -> (13.9373, 44.5553) centre (8.2554, 42.6182) ccw
  arc A13 (13.9373, 44.5553) -> (13.436, 44.5913) centre (13, 35.0012) ccw
  arc A14 (13.436, 44.5913) -> (12.9429, 43.251) centre (18.7832, 41.8629) ccw
  arc A15 (12.9429, 43.251) -> (12.5112, 43.2367) centre (13, 35.0012) ccw
  arc A16 (12.5112, 43.2367) -> (11.9304, 44.5414) centre (6.7755, 41.4653) ccw
  arc A17 (11.9304, 44.5414) -> (11.4326, 44.4724) centre (13, 35.0012) ccw
  arc A18 (11.4326, 44.4724) -> (11.2289, 43.0588) centre (17.2302, 42.9154) ccw
  arc A19 (11.2289, 43.0588) -> (10.8096, 42.9551) centre (13, 35.0012) ccw
  arc A20 (10.8096, 42.9551) -> (9.9703, 44.1106) centre (5.5675, 40.0299) ccw
  arc A21 (9.9703, 44.1106) -> (9.4977, 43.9395) centre (13, 35.0012) ccw
  arc A22 (9.4977, 43.9395) -> (9.5923, 42.5145) centre (15.4923, 43.622) ccw
  arc A23 (9.5923, 42.5145) -> (9.2038, 42.3259) centre (13, 35.0012) ccw
  arc A24 (9.2038, 42.3259) -> (8.1425, 43.2816) centre (4.6844, 38.3747) ccw
  arc A25 (8.1425, 43.2816) -> (7.7158, 43.016) centre (13, 35.0012) ccw
  arc A26 (7.7158, 43.016) -> (8.1047, 41.6418) centre (13.6455, 43.9518) ccw
  arc A27 (8.1047, 41.6418) -> (7.7638, 41.3765) centre (13, 35.0012) ccw
  arc A28 (7.7638, 41.3765) -> (6.5271, 42.0907) centre (4.1648, 36.572) ccw
  arc A29 (6.5271, 42.0907) -> (6.1649, 41.7423) centre (13, 35.0012) ccw
  arc A30 (6.1649, 41.7423) -> (6.831, 40.4789) centre (11.7705, 43.8904) ccw
  arc A31 (6.831, 40.4789) -> (6.5527, 40.1486) centre (13, 35.0012) ccw
  arc A32 (6.5527, 40.1486) -> (5.1945, 40.59) centre (4.0312, 34.7008) ccw
  arc A33 (5.1945, 40.59) -> (4.9127, 40.1739) centre (13, 35.0012) ccw
  arc A34 (4.9127, 40.1739) -> (5.8269, 39.0766) centre (9.9492, 43.4405) ccw
  arc A35 (5.8269, 39.0766) -> (5.6234, 38.6956) centre (13, 35.0012) ccw
  arc A36 (5.6234, 38.6956) -> (4.2031, 38.845) centre (4.2897, 32.8426) ccw
  arc A37 (4.2031, 38.845) -> (4.014, 38.3794) centre (13, 35.0012) ccw
  arc A38 (4.014, 38.3794) -> (5.1363, 37.4962) centre (8.2612, 42.6218) ccw
  arc A39 (5.1363, 37.4962) -> (5.0165, 37.0812) centre (13, 35.0012) ccw
  arc A40 (5.0165, 37.0812) -> (3.5962, 36.9321) centre (4.9288, 31.0788) ccw
  arc A41 (3.5962, 36.9321) -> (3.508, 36.4373) centre (13, 35.0012) ccw
  arc A42 (3.508, 36.4373) -> (4.7894, 35.8067) centre (6.7804, 41.47) ccw
  arc A43 (4.7894, 35.8067) -> (4.7585, 35.3759) centre (13, 35.0012) ccw
  arc A44 (4.7585, 35.3759) -> (3.4002, 34.9347) centre (5.9207, 29.4864) ccw
  arc A45 (3.4002, 34.9347) -> (3.4169, 34.4324) centre (13, 35.0012) ccw
  arc A46 (3.4169, 34.4324) -> (4.8014, 34.082) centre (5.5713, 40.0355) ccw
  arc A47 (4.8014, 34.082) -> (4.8607, 33.6542) centre (13, 35.0012) ccw
  arc A48 (4.8607, 33.6542) -> (3.6238, 32.9403) centre (7.222, 28.1351) ccw
  arc A49 (3.6238, 32.9403) -> (3.7445, 32.4524) centre (13, 35.0012) ccw
  arc A50 (3.7445, 32.4524) -> (5.1716, 32.3975) centre (4.687, 38.381) ccw
  arc A51 (5.1716, 32.3975) -> (5.3186, 31.9914) centre (13, 35.0012) ccw
  arc A52 (5.3186, 31.9914) -> (4.2572, 31.0359) centre (8.7758, 27.0838) ccw
  arc A53 (4.2572, 31.0359) -> (4.4767, 30.5838) centre (13, 35.0012) ccw
  arc A54 (4.4767, 30.5838) -> (5.884, 30.8268) centre (4.1659, 36.5788) ccw
  arc A55 (5.884, 30.8268) -> (6.1122, 30.4601) centre (13, 35.0012) ccw
  arc A56 (6.1122, 30.4601) -> (5.2727, 29.3048) centre (10.5142, 26.3786) ccw
  arc A57 (5.2727, 29.3048) -> (5.5814, 28.9082) centre (13, 35.0012) ccw
  arc A58 (5.5814, 28.9082) -> (6.9074, 29.4385) centre (4.031, 34.7076) ccw
  arc A59 (6.9074, 29.4385) -> (7.2069, 29.1273) centre (13, 35.0012) ccw
  arc A60 (7.2069, 29.1273) -> (6.6259, 27.8227) centre (12.3613, 26.0502) ccw
  arc A61 (6.6259, 27.8227) -> (7.0103, 27.4989) centre (13, 35.0012) ccw
  arc A62 (7.0103, 27.4989) -> (8.1971, 28.2934) centre (4.288, 32.8492) ccw
  arc A63 (8.1971, 28.2934) -> (8.5548, 28.0512) centre (13, 35.0012) ccw
  arc A64 (8.5548, 28.0512) -> (8.2577, 26.6543) centre (14.2363, 26.113) ccw
  arc A65 (8.2577, 26.6543) -> (8.701, 26.4176) centre (13, 35.0012) ccw
  arc A66 (8.701, 26.4176) -> (9.6967, 27.4414) centre (4.9258, 31.0849) ccw
  arc A67 (9.6967, 27.4414) -> (10.0969, 27.2789) centre (13, 35.0012) ccw
  arc A68 (10.0969, 27.2789) -> (10.0967, 25.8507) centre (16.0572, 26.5642) ccw
  arc A69 (10.0967, 25.8507) -> (10.5796, 25.7113) centre (13, 35.0012) ccw
  arc A70 (10.5796, 25.7113) -> (11.3407, 26.9198) centre (5.9165, 29.4918) ccw
  arc A71 (11.3407, 26.9198) -> (11.7659, 26.844) centre (13, 35.0012) ccw
  arc A72 (11.7659, 26.844) -> (12.0627, 25.4471) centre (17.7446, 27.3842) ccw
  arc A73 (12.0627, 25.4471) -> (12.564, 25.4111) centre (13, 35.0012) ccw
  arc A74 (12.564, 25.4111) -> (13.0571, 26.7514) centre (7.2168, 28.1395) ccw
  arc A75 (13.0571, 26.7514) -> (13.4888, 26.7657) centre (13, 35.0012) ccw
  arc A76 (13.4888, 26.7657) -> (14.0696, 25.461) centre (19.2245, 28.5371) ccw
  arc A77 (14.0696, 25.461) -> (14.5674, 25.53) centre (13, 35.0012) ccw
  arc A78 (14.5674, 25.53) -> (14.7711, 26.9436) centre (8.7698, 27.087) ccw
  arc A79 (14.7711, 26.9436) -> (15.1904, 27.0473) centre (13, 35.0012) ccw
  arc A80 (15.1904, 27.0473) -> (16.0297, 25.8918) centre (20.4325, 29.9725) ccw
  arc A81 (16.0297, 25.8918) -> (16.5023, 26.0629) centre (13, 35.0012) ccw
  arc A82 (16.5023, 26.0629) -> (16.4077, 27.4879) centre (10.5077, 26.3804) ccw
  arc A83 (16.4077, 27.4879) -> (16.7962, 27.6765) centre (13, 35.0012) ccw
  arc A84 (16.7962, 27.6765) -> (17.8575, 26.7208) centre (21.3156, 31.6277) ccw
  arc A85 (17.8575, 26.7208) -> (18.2842, 26.9864) centre (13, 35.0012) ccw
  arc A86 (18.2842, 26.9864) -> (17.8953, 28.3605) centre (12.3545, 26.0506) ccw
  arc A87 (17.8953, 28.3605) -> (18.2362, 28.6259) centre (13, 35.0012) ccw
  arc A88 (18.2362, 28.6259) -> (19.4729, 27.9117) centre (21.8352, 33.4304) ccw
  arc A89 (19.4729, 27.9117) -> (19.8351, 28.2601) centre (13, 35.0012) ccw
  arc A90 (19.8351, 28.2601) -> (19.169, 29.5235) centre (14.2295, 26.112) ccw
  arc A91 (19.169, 29.5235) -> (19.4473, 29.8538) centre (13, 35.0012) ccw
  arc A92 (19.4473, 29.8538) -> (20.8055, 29.4124) centre (21.9688, 35.3016) ccw
  arc A93 (20.8055, 29.4124) -> (21.0873, 29.8285) centre (13, 35.0012) ccw
  arc A94 (21.0873, 29.8285) -> (20.1731, 30.9258) centre (16.0508, 26.5619) ccw
  arc A95 (20.1731, 30.9258) -> (20.3766, 31.3068) centre (13, 35.0012) ccw
  arc A96 (20.3766, 31.3068) -> (21.7969, 31.1574) centre (21.7103, 37.1598) ccw
  arc A97 (21.7969, 31.1574) -> (21.986, 31.623) centre (13, 35.0012) ccw
  arc A98 (21.986, 31.623) -> (20.8637, 32.5062) centre (17.7388, 27.3806) ccw
  arc A99 (20.8637, 32.5062) -> (20.9835, 32.9212) centre (13, 35.0012) ccw
  arc A100 (20.9835, 32.9212) -> (22.4038, 33.0703) centre (21.0712, 38.9236) ccw
  arc A101 (22.4038, 33.0703) -> (22.492, 33.5651) centre (13, 35.0012) ccw
  arc A102 (22.492, 33.5651) -> (21.2106, 34.1957) centre (19.2196, 28.5324) ccw
  arc A103 (21.2106, 34.1957) -> (21.2415, 34.6265) centre (13, 35.0012) ccw
  arc A104 (21.2415, 34.6265) -> (22.5998, 35.0677) centre (20.0793, 40.516) ccw
  arc A105 (22.5998, 35.0677) -> (22.5831, 35.57) centre (13, 35.0012) ccw
  arc A106 (22.5831, 35.57) -> (21.1986, 35.9204) centre (20.4287, 29.9669) ccw
  arc A107 (21.1986, 35.9204) -> (21.1393, 36.3482) centre (13, 35.0012) ccw
  arc A108 (21.1393, 36.3482) -> (22.3762, 37.0621) centre (18.778, 41.8673) ccw
  arc A109 (22.3762, 37.0621) -> (22.2555, 37.55) centre (13, 35.0012) ccw
  arc A110 (22.2555, 37.55) -> (20.8284, 37.6049) centre (21.313, 31.6214) ccw
  arc A111 (20.8284, 37.6049) -> (20.6814, 38.011) centre (13, 35.0012) ccw
  arc A112 (20.6814, 38.011) -> (21.7428, 38.9665) centre (17.2242, 42.9186) ccw
  arc A113 (21.7428, 38.9665) -> (21.5233, 39.4186) centre (13, 35.0012) ccw
  arc A114 (21.5233, 39.4186) -> (20.116, 39.1756) centre (21.8341, 33.4236) ccw
  arc A115 (20.116, 39.1756) -> (19.8878, 39.5423) centre (13, 35.0012) ccw
  arc A116 (19.8878, 39.5423) -> (20.7273, 40.6976) centre (15.4858, 43.6238) ccw
  arc A117 (20.7273, 40.6976) -> (20.4186, 41.0942) centre (13, 35.0012) ccw
  arc A118 (20.4186, 41.0942) -> (19.0926, 40.5639) centre (21.969, 35.2948) ccw
  arc A119 (19.0926, 40.5639) -> (18.7931, 40.8751) centre (13, 35.0012) ccw
  circle A120 centre (14.5, 55.2958) radius 14.5
  circle A121 centre (14.5, 55.2958) radius 13.85
  line L20 (23.8, 65.2958) -> (27, 65.2958)
  line L21 (23.8, 69.2958) -> (27, 69.2958)
  point P0 (0, 0)
  point P1 (5.0862, 65.2958)
  point P2 (4, 65.2958)
  point P3 (4.0351, 65.3325)
  point P4 (4.9176, 65.2958)
  point P5 (4.9235, 65.3015)
extrude "Extrusion7" add sketch "Sketch4" along normal blind 14.5 contours L20 A121 L3 A120 | A120 L3 L21 L15 L20 | L20 L3 A121 | A120 L4 L3 | L3 A121 L2 A120 L4 | L21 L4 A120 L5 L6 L7 L16 L15 | L3 L13 L2 A121 | L4 A120 | A120 L2 L14 L12 L11 L10 L9 L8 L7 L6 L5 L4
ref_plane "Work Plane4" through (-23.1368, 52.6716, -30.5) normal (0, 0, 1) x (0.9993908, 0.0348995, 0)
extrude "Extrusion8" add sketch "Sketch4" against normal up to surface (5 mm away) contours L20 A121 L3 A120 | A120 L3 L21 L15 L20 | L20 L3 A121
ref_plane "Work Plane5" through (-23.1368, 52.6716, -30.5) normal (0, 0, 1) x (0.9993908, 0.0348995, 0)
extrude "Extrusion9" cut sketch "Sketch4" against normal up to surface (5 mm away) contours L13 A120 L2 | A120 L13 L12 L14 L2